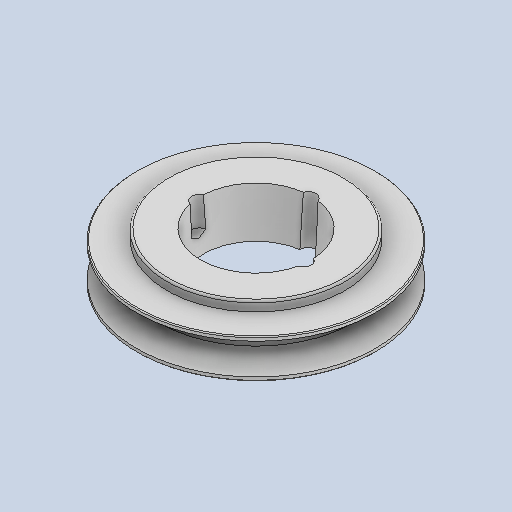
# Autodesk Inventor part: Шкив 118 мм
Saved by Autodesk Inventor 2025 (Build 290162010, 162A)
## iProperties
Created: 2024-04-08
Part Number: Шкив 118 мм
Material: Generic
Document SubType Name: Modeling
Designer: pokla
Density: 1 g/cm^3
Appearance: Default
Stock Number: Шкив 118 мм
Author: pokla
Autodesk Inventor part; units mm, degrees
ref_plane "YZ Plane" through (0, 0, 0) normal (1, 0, 0) x (0, 1, 0)
ref_plane "XZ Plane" through (0, 0, 0) normal (0, 1, 0) x (-1, 0, 0)
ref_plane "XY Plane" through (0, 0, 0) normal (0, 0, 1) x (1, 0, 0)
sketch "Sketch1" plane through (0, 0, 0) normal (1, 0, 0) x (0, 1, 0)
  line L0 (25, -28.535) -> (25, -46)
  line L1 (25, -46) -> (20, -46)
  line L2 (20, -46) -> (20, -61.75)
  line L3 (20, -61.75) -> (18, -61.75)
  line L4 (18, -61.75) -> (12.5, -50)
  line L5 (12.5, -50) -> (7.5, -50)
  line L6 (2, -61.75) -> (0, -61.75)
  line L7 (7.5, -50) -> (2, -61.75)
  line L8 (-5, 0) -> (30, 0) projected
  line L9 (0, -61.75) -> (0, -26.985)
  line L10 (25, -28.535) -> (0, -26.985)
  point P0 (0, 0)
  point P1 (10, -50)
  dimension "d4" = 5
  dimension "d5" = 2
  dimension "d24" = 28.535
  dimension "d26" = 5
  dimension "d27" = 17.465
  dimension "d29" = 26.985
  dimension "d30" = 61.75
  dimension "d31" = 25
  dimension "d32" = 50
  constraints: 20 end point, 4 perpendicular, 2 equal length, 2 point on line, 1 midpoint, 1 vertical, 1 vertical alignment
  measures "d4" distance of L4.end L5.end
  measures "d5" distance of L6.start L6.end
  measures "d24" vertical distance of point (0, 0) L0.start
  measures "d26" distance of L0.end L1.end
  measures "d27" distance of L0.start L0.end
  measures "d29" distance of point (0, 0) L9.end
  measures "d30" distance of L6.end point (0, 0)
  measures "d31" distance between parallel lines of L0 L9
  measures "d32" vertical distance of point (0, 0) point (10, -50)
revolve "Revolution1" add sketch "Sketch1" angle 360 about axis through (0, -10, 0) along (0, 1, 0)
fillet "Fillet1" radius 1 1 edges at (0, 25, 46)
fillet "Fillet2" radius 0.5 2 edges at (0, 20, 61.75) (0, 0, 61.75)
sketch "Sketch5" plane through (0, 25, 0) normal (0, 1, 0) x (1, 0, 0)
  circle A0 centre (0, 0) radius 26.985 projected
  line L0 (0, 0) -> (0, 26.985) construction
  constraints: 2 end point, 1 coincident, 1 vertical, 1 vertical alignment, 1 other
hole "Hole1" at (0, 25, -26.985) direction (0, -1, 0) diameter 8 end through all
sketch "Sketch6" plane through (0, 25, 0) normal (0, 1, 0) x (1, 0, 0)
  line L0 (0, 0) -> (26.8823, -2.3519) construction
  arc A0 (-3.989, 26.6885) -> (3.989, 26.6885) centre (0, 0) ccw projected
  line L1 (0, 0) -> (0, -26.985) construction
  line L2 (0, 0) -> (-26.8823, -2.3519) construction
  dimension "d40" = 85
  dimension "d41" = 85
  constraints: 6 end point, 3 point on circle, 2 coincident
  measures "d40" angle of L1 L0
  measures "d41" angle of L2 L1
hole "Hole2" at (26.8823, 25, 2.3519) at (-26.8823, 25, 2.3519) direction (0, -1, 0) diameter 8 depth 15 tip angle 118
equation "\"d41\" = d40"
body "Solid1"
